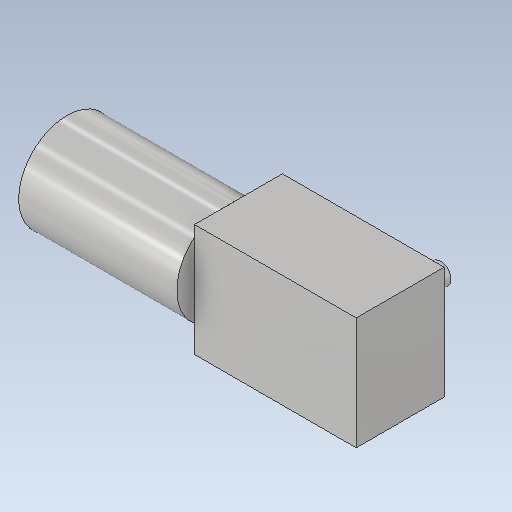
# Autodesk Inventor part: motor
Saved by Autodesk Inventor 2020 (Build 240168000, 168)
## iProperties
Created: 2017-11-25
Part Number: motor
Material: Generic
Document SubType Name: Modeling
Designer: stedrock
Density: 1 g/cm^3
Appearance: Default
Mass: 63.7225 g
Surface Area: 113.743 cm^2
Volume: 63.7225 cm^3
Author: stedrock
Autodesk Inventor part; units mm, degrees
ref_plane "YZ Plane" through (0, 0, 0) normal (1, 0, 0) x (0, 1, 0)
ref_plane "XZ Plane" through (0, 0, 0) normal (0, 1, 0) x (-1, 0, 0)
ref_plane "XY Plane" through (0, 0, 0) normal (0, 0, 1) x (1, 0, 0)
sketch "Sketch1" plane through (0, 0, 0) normal (0, 0, 1) x (1, 0, 0)
  line L0 (23, -16) -> (-23, -16)
  line L1 (-23, -16) -> (-23, 16)
  line L2 (-23, 16) -> (23, 16)
  line L3 (23, 16) -> (23, -16)
  line L4 (23, -16) -> (-23, 16) construction
  line L5 (-23, -16) -> (23, 16) construction
  line L6 (0, 0) -> (32.2248, 0) construction
  line L7 (0, 0) -> (0, 21.3704) construction
  circle A0 centre (8, 0) radius 3
  circle A1 centre (17, 9) radius 1.5
  circle A2 centre (-16, 9) radius 1.5
  line L8 (17, 9) -> (-16, 9) construction
  circle A3 centre (17, -9) radius 1.5
  circle A4 centre (-16, -9) radius 1.5
  line L9 (5.7769, -2.0144) -> (5.7769, 2.0144)
  dimension "d0" = 46
  dimension "d1" = 32
  dimension "d2" = 6
  dimension "d3" = 15
  dimension "d7" = 3
  dimension "d9" = 3
  dimension "d14" = 33
  dimension "d15" = 9
  dimension "d16" = 9
  constraints: 20 end point, 5 centre point, 3 parallel, 2 horizontal, 2 midpoint, 2 point on circle, 2 symmetric about line, 2 vertical, 1 coincident, 1 perpendicular, 1 point on line, 2 other
  measures "d0" distance of L1.end L2.end
  measures "d1" distance of L0.end L1.end
  measures "d2" diameter of A0
  measures "d3" distance from line of L3 A0.centre
  measures "d7" diameter of A1
  measures "d9" diameter of A2
  measures "d14" distance of A2.centre L8.start
  measures "d15" distance from line of L6 L8.start
  measures "d16" horizontal distance of A0.centre L8.start
extrude "Extrusion1" add sketch "Sketch1" against normal blind 14 contours A0 L9 picked at (7.5179, 0)
extrude "Extrusion2" add sketch "Sketch1" against normal blind 2.5 contours A0 L9 | L9 A0
extrude "Extrusion3" add sketch "Sketch1" along normal blind 25 contours L0 L1 L2 L3 | A0 L9 | L9 A0 | A1 | A2 | A3 | A4
extrude "Extrusion4" cut sketch "Sketch1" along normal blind 5 contours A1 | A2 | A3 | A4
sketch "Sketch2" plane through (-23, -16, 0) normal (-1, 0, 0) x (0, 0, 1)
  circle A0 centre (16.25, 18.25) radius 13.75
  line L0 (0, 32) -> (25, 32) projected
  line L1 (0, 0) -> (0, 32) projected
  point P0 (0, 16)
  dimension "d23" = 27.5
  dimension "d24" = 16.25
  constraints: 1 centre point, 1 tangent
  measures "d23" diameter of A0
  measures "d24" distance from line of A0.centre L1
extrude "Extrusion5" add sketch "Sketch2" along normal blind 45
sketch "Sketch3" plane through (0, 0, -14) normal (0, 0, -1) x (-1, 0, 0)
  arc A0 (-5.7769, 2.0144) -> (-5.7769, -2.0144) centre (-8, 0) ccw projected
  circle A1 centre (-8, 0) radius 1.5
  point P0 (0, 0)
  dimension "d29" = 3
  constraints: 1 centre point, 1 coincident
  measures "d29" diameter of A1
extrude "Extrusion7" cut sketch "Sketch3" against normal blind 5
body "Solid2"
